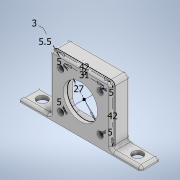
# Autodesk Inventor part: stepper_mount
Saved by Autodesk Inventor 2021 (Build 250183000, 183)
## iProperties
Created: 2021-06-16
Part Number: stepper_mount
Material: Generic
Document SubType Name: Modeling
Designer: Charlie
Density: 1 g/cm^3
Appearance: Default
Author: Charlie
Autodesk Inventor part; units mm, degrees
ref_plane "YZ Plane" through (0, 0, 0) normal (1, 0, 0) x (0, 1, 0)
ref_plane "XZ Plane" through (0, 0, 0) normal (0, 1, 0) x (-1, 0, 0)
ref_plane "XY Plane" through (0, 0, 0) normal (0, 0, 1) x (1, 0, 0)
sketch "Sketch1" plane through (0, 0, 0) normal (0, 0, 1) x (1, 0, 0)
  line L0 (-15.5, -21) -> (15.5, -21)
  line L1 (21, -15.5) -> (21, 15.5)
  line L2 (15.5, 21) -> (-15.5, 21)
  line L3 (-21, 15.5) -> (-21, -15.5)
  line L4 (-21, -21) -> (21, 21) construction
  line L5 (21, -21) -> (-21, 21) construction
  line L6 (-15.5, -14.7483) -> (15.5, -14.7483) construction
  line L7 (15.5, -14.7483) -> (15.5, 14.7483) construction
  line L8 (15.5, 14.7483) -> (-15.5, 14.7483) construction
  line L9 (-15.5, 14.7483) -> (-15.5, -14.7483) construction
  line L10 (-15.5, -14.7483) -> (15.5, 14.7483) construction
  line L11 (15.5, -14.7483) -> (-15.5, 14.7483) construction
  circle A0 centre (-15.5, 14.7483) radius 2.5
  circle A1 centre (15.5, 14.7483) radius 2.5
  circle A2 centre (15.5, -14.7483) radius 2.5
  circle A3 centre (-15.5, -14.7483) radius 2.5
  circle A4 centre (0, 0) radius 13.5
  line L12 (-21, 24) -> (21, 24)
  line L13 (24, 21) -> (24, -24)
  line L14 (24, -24) -> (-24, -24)
  line L15 (-24, -24) -> (-24, 21)
  arc A5 (-15.5, 21) -> (-21, 15.5) centre (-15.5, 15.5) ccw
  arc A6 (21, 15.5) -> (15.5, 21) centre (15.5, 15.5) ccw
  arc A7 (15.5, -21) -> (21, -15.5) centre (15.5, -15.5) ccw
  arc A8 (-21, -15.5) -> (-15.5, -21) centre (-15.5, -15.5) ccw
  arc A9 (-21, 24) -> (-24, 21) centre (-21, 21) ccw
  arc A10 (24, 21) -> (21, 24) centre (21, 21) ccw
  dimension "d0" = 42
  dimension "d1" = 42
  dimension "d2" = 31
  dimension "d3" = 5
  dimension "d4" = 5
  dimension "d5" = 5
  dimension "d6" = 5
  dimension "d7" = 27
  dimension "d8" = 3
  dimension "d9" = 5.5
  dimension "d10" = 3
  constraints: 32 end point, 12 point on circle, 12 tangent, 11 centre point, 8 point on line, 6 parallel, 5 coincident, 4 equal radius, 4 midpoint, 3 perpendicular, 2 horizontal, 3 other
  measures "d0" distance of L5.end L4.end
  measures "d1" distance of L4.end L5.start
  measures "d2" distance of L8.end L7.end
  measures "d3" diameter of A0
  measures "d4" diameter of A1
  measures "d5" diameter of A2
  measures "d6" diameter of A3
  measures "d7" diameter of A4
  measures "d8" distance between parallel lines of L2 L12
  measures "d9" radius of A5
  measures "d10" radius of A9
extrude "Extrusion1" add sketch "Sketch1" along normal blind 3 contours A8 L3 A5 L2 A6 L1 A7 L0 | L12 A10 L13 L14 L15 A9
extrude "Extrusion2" add sketch "Sketch1" against normal blind 12 contours L12 A10 L13 L14 L15 A9
sketch "Sketch2" plane through (-24, -24, 3) normal (0, -1, 0) x (1, 0, 0)
  circle A0 centre (61.5, -7.5) radius 4
  circle A1 centre (-13.5, -7.5) radius 4
  line L0 (71.5, 0) -> (-23.5, 0)
  line L1 (-23.5, 0) -> (-23.5, -15)
  line L2 (-23.5, -15) -> (71.5, -15)
  line L3 (71.5, -15) -> (71.5, 0)
  line L4 (71.5, 0) -> (-23.5, -15) construction
  line L5 (-23.5, 0) -> (71.5, -15) construction
  point P0 (24, -3)
  point P1 (24, -7.5)
  dimension "d15" = 8
  dimension "d16" = 8
  dimension "d17" = 95
  dimension "d18" = 15
  dimension "d21" = 37.5
  dimension "d22" = 37.5
  constraints: 12 end point, 2 centre point, 2 midpoint, 2 parallel, 1 horizontal, 1 perpendicular
  measures "d15" diameter of A0
  measures "d16" diameter of A1
  measures "d17" distance of L2.end L1.end
  measures "d18" distance of L1.end L0.end
  measures "d21" distance of point (24, -7.5) A0.centre
  measures "d22" distance of A1.centre point (24, -7.5)
extrude "Extrusion3" add sketch "Sketch2" against normal blind 3
fillet "Fillet1" radius 2 20 edges at (47.5, -22.5, -12) (47.5, -22.5, 3) (24, -21, -4.5) (-23.1213, 23.1213, -12) (0, 24, -12) (23.1213, 23.1213, -12) (24, 0, -12) (-24, 0, -12) (-24, -21, -4.5) (-23.1213, 23.1213, 3) (0, 24, 3) (23.1213, 23.1213, 3) (24, 0, 3) (-24, 0, 3) (-47.5, -21, -4.5) (-35.75, -21, -12) (-35.75, -21, 3) (35.75, -21, -12) (35.75, -21, 3) (47.5, -21, -4.5)
body "Solid1"
